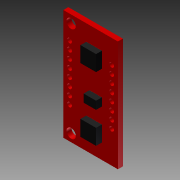
# Autodesk Inventor part: IMU
Saved by Autodesk Inventor 2012 (Build 160160000, 160)
## iProperties
Created: 2012-03-02
Part Number: IMU
Material: Default
Document SubType Name: Modeling
Designer: Lauszus
Density: 1 g/cm^3
Author: Lauszus
Autodesk Inventor part; units mm, degrees
ref_plane "YZ Plane" through (0, 0, 0) normal (1, 0, 0) x (0, 1, 0)
ref_plane "XZ Plane" through (0, 0, 0) normal (0, 1, 0) x (-1, 0, 0)
ref_plane "XY Plane" through (0, 0, 0) normal (0, 0, 1) x (1, 0, 0)
sketch "Sketch1" plane through (0, 0, 0) normal (0, 0, 1) x (1, 0, 0)
  line L0 (35.093, -7.2202) -> (-19.907, -7.2202)
  line L1 (-19.907, -7.2202) -> (-19.907, 74.7798)
  line L2 (-19.907, 74.7798) -> (35.093, 74.7798)
  line L3 (35.093, 74.7798) -> (35.093, -7.2202)
  line L4 (-1.6316, 73.7798) -> (15.8684, 73.7798)
  line L5 (15.8684, 73.7798) -> (15.8684, 38.2798)
  line L6 (15.8684, 38.2798) -> (-1.6316, 38.2798)
  line L7 (-1.6316, 38.2798) -> (-1.6316, 73.7798)
  circle A0 centre (7.5885, 28.2798) radius 5.75
  line L8 (12.233, 6.0025) -> (3.233, 6.0025)
  line L9 (3.233, 6.0025) -> (3.233, -3.9975)
  line L10 (3.233, -3.9975) -> (12.233, -3.9975)
  line L11 (12.233, -3.9975) -> (12.233, 6.0025)
  circle A1 centre (7.5885, 28.2798) radius 1.25
  line L12 (3.233, 6.0025) -> (-2.767, 6.0025)
  line L13 (-2.767, 6.0025) -> (-2.767, -3.9975)
  line L14 (-2.767, -3.9975) -> (3.233, -3.9975)
  line L15 (3.233, -3.9975) -> (3.233, 6.0025)
  line L16 (12.233, 5.3167) -> (16.7288, 5.3167)
  line L17 (16.7288, 5.3167) -> (16.7288, 2.7767)
  line L18 (16.7288, 2.7767) -> (12.233, 2.7767)
  line L19 (12.233, 2.7767) -> (12.233, 5.3167)
  line L20 (12.233, -1.5375) -> (12.233, 1.0025)
  line L21 (12.233, -3.4895) -> (12.233, -0.9495)
  line L22 (12.233, 2.2687) -> (16.7288, 2.2687)
  line L23 (16.7288, 2.2687) -> (16.7288, -0.2713)
  line L24 (16.7288, -0.2713) -> (12.233, -0.2713)
  line L25 (12.233, -0.2713) -> (12.233, 2.2687)
  line L26 (12.233, -0.7793) -> (16.7288, -0.7793)
  line L27 (16.7288, -0.7793) -> (16.7288, -3.3193)
  line L28 (16.7288, -3.3193) -> (12.233, -3.3193)
  line L29 (12.233, -3.3193) -> (12.233, -0.7793)
  circle A2 centre (0.233, 0.9987) radius 1.5
  circle A3 centre (0.3684, 66.2798) radius 0.75
  circle A4 centre (0.3684, 63.7398) radius 0.75
  circle A5 centre (0.3684, 61.1998) radius 0.75
  circle A6 centre (0.3684, 58.6598) radius 0.75
  circle A7 centre (0.3684, 56.1198) radius 0.75
  circle A8 centre (0.3684, 53.5798) radius 0.75
  circle A9 centre (0.3684, 51.0398) radius 0.75
  circle A10 centre (0.3684, 48.4998) radius 0.75
  circle A11 centre (13.8684, 63.7398) radius 0.75
  circle A12 centre (13.8684, 58.6598) radius 0.75
  circle A13 centre (13.8684, 56.1198) radius 0.75
  circle A14 centre (13.8684, 53.5798) radius 0.75
  circle A15 centre (13.8684, 48.4998) radius 0.75
  circle A16 centre (13.8684, 66.2798) radius 0.75
  circle A17 centre (13.8684, 51.0398) radius 0.75
  circle A18 centre (13.8684, 61.1998) radius 0.75
  line L30 (-17.907, 69.7798) -> (-16.407, 69.7798)
  line L31 (-16.407, 69.7798) -> (-16.407, -2.2202)
  line L32 (-16.407, -2.2202) -> (-17.907, -2.2202)
  line L33 (-17.907, -2.2202) -> (-17.907, 69.7798)
  line L34 (-15.367, -2.2202) -> (-13.867, -2.2202)
  line L35 (-13.867, -2.2202) -> (-13.867, 69.7798)
  line L36 (-13.867, 69.7798) -> (-15.367, 69.7798)
  line L37 (-15.367, 69.7798) -> (-15.367, -2.2202)
  line L38 (31.593, 69.7798) -> (33.093, 69.7798)
  line L39 (33.093, 69.7798) -> (33.093, -2.2202)
  line L40 (33.093, -2.2202) -> (31.593, -2.2202)
  line L41 (31.593, -2.2202) -> (31.593, 69.7798)
  line L42 (30.553, -2.2202) -> (29.053, -2.2202)
  line L43 (29.053, -2.2202) -> (29.053, 69.7798)
  line L44 (29.053, 69.7798) -> (30.553, 69.7798)
  line L45 (30.553, 69.7798) -> (30.553, -2.2202)
  line L46 (5.8684, 68.7798) -> (10.8684, 68.7798)
  line L47 (10.8684, 68.7798) -> (10.8684, 63.7798)
  line L48 (10.8684, 63.7798) -> (5.8684, 63.7798)
  line L49 (5.8684, 63.7798) -> (5.8684, 68.7798)
  line L50 (6.8684, 55.8198) -> (10.8684, 55.8198)
  line L51 (10.8684, 55.8198) -> (10.8684, 53.2798)
  line L52 (10.8684, 53.2798) -> (6.8684, 53.2798)
  line L53 (6.8684, 53.2798) -> (6.8684, 55.8198)
  line L54 (5.8684, 48.2798) -> (10.8684, 48.2798)
  line L55 (10.8684, 48.2798) -> (10.8684, 43.2798)
  line L56 (10.8684, 43.2798) -> (5.8684, 43.2798)
  line L57 (5.8684, 43.2798) -> (5.8684, 48.2798)
  circle A19 centre (0.8684, 71.2798) radius 1.5
  circle A20 centre (0.8684, 40.7798) radius 1.5
  point P0 (0, 0)
  point P1 (0, 0)
  dimension "d0" = 82
  dimension "d1" = 55
  dimension "d2" = 17.5
  dimension "d3" = 35.5
  dimension "d4" = 11.5
  dimension "d5" = 2.5
  dimension "d6" = 1
  dimension "d7" = 10
  dimension "d8" = 27.4955
  dimension "d9" = 9
  dimension "d10" = 10
  dimension "d11" = 6
  dimension "d12" = 22.86
  dimension "d13" = 19.2246
  dimension "d14" = 2.54
  dimension "d15" = 0.6858
  dimension "d16" = 10
  dimension "d17" = 2.54
  dimension "d18" = 0.508
  dimension "d19" = 4.4958
  dimension "d20" = 4.4958
  dimension "d21" = 2.54
  dimension "d22" = 4.4958
  dimension "d23" = 0.508
  dimension "d24" = 3
  dimension "d25" = 1.5
  dimension "d26" = 7.5
  dimension "d27" = 2
  dimension "d28" = 1.5
  dimension "d29" = 1.5
  dimension "d30" = 1.5
  dimension "d31" = 1.5
  dimension "d32" = 1.5
  dimension "d33" = 1.5
  dimension "d34" = 1.5
  dimension "d35" = 2.54
  dimension "d36" = 2.54
  dimension "d37" = 2.54
  dimension "d38" = 2.54
  dimension "d39" = 2.54
  dimension "d40" = 2.54
  dimension "d41" = 2.54
  dimension "d42" = 1.5
  dimension "d43" = 1.5
  dimension "d44" = 1.5
  dimension "d45" = 1.5
  dimension "d46" = 1.5
  dimension "d47" = 1.5
  dimension "d48" = 1.5
  dimension "d49" = 1.5
  dimension "d50" = 2.54
  dimension "d51" = 2.54
  dimension "d52" = 2.54
  dimension "d53" = 2.54
  dimension "d54" = 2.54
  dimension "d55" = 2.54
  dimension "d56" = 2.54
  dimension "d57" = 2
  dimension "d58" = 7.5
  dimension "d59" = 2
  dimension "d60" = 2
  dimension "d61" = 2
  dimension "d62" = 2
  dimension "d63" = 2
  constraints: 116 end point, 28 parallel, 21 centre point, 14 horizontal, 14 perpendicular, 4 point on line, 1 coincident, 1 midpoint
  measures "d0" distance of L0.end L1.end
  measures "d1" distance of L1.end L2.end
  measures "d2" distance of L4.start L4.end
  measures "d3" distance of L4.end L5.end
  measures "d4" diameter of A0
  measures "d5" diameter of A1
  measures "d6" distance between parallel lines of L2 L4
  measures "d7" distance from line of A0.centre L6
  measures "d8" distance from line of L1 A0.centre
  measures "d9" distance between parallel lines of L9 L11
  measures "d10" distance of L10.end L8.start
  measures "d11" distance of L8.end L12.end
  measures "d12" distance between parallel lines of L3 L11
  measures "d13" distance between parallel lines of L3 L5
  measures "d14" distance of L16.end L17.end
  measures "d15" distance between parallel lines of L8 L16
  measures "d16" distance of L14.end L8.end
  measures "d17" distance of L22.end L23.end
  measures "d18" distance between parallel lines of L18 L22
  measures "d19" distance of L16.start L16.end
  measures "d20" distance of L22.start L22.end
  measures "d21" distance of L26.end L27.end
  measures "d22" distance of L26.start L26.end
  measures "d23" distance between parallel lines of L24 L26
  measures "d24" diameter of A2
  measures "d25" diameter of A3
  measures "d26" distance from line of L4 A3.centre
  measures "d27" distance from line of L7 A3.centre
  measures "d28" diameter of A4
  measures "d29" diameter of A5
  measures "d30" diameter of A6
  measures "d31" diameter of A7
  measures "d32" diameter of A8
  measures "d33" diameter of A9
  measures "d34" diameter of A10
  measures "d35" distance of A4.centre A3.centre
  measures "d36" distance between centres of A5 A4
  measures "d37" distance between centres of A6 A5
  measures "d38" distance of A7.centre A6.centre
  measures "d39" distance between centres of A8 A7
  measures "d40" distance between centres of A9 A8
  measures "d41" distance between centres of A10 A9
  measures "d42" diameter of A16
  measures "d43" diameter of A11
  measures "d44" diameter of A18
  measures "d45" diameter of A12
  measures "d46" diameter of A13
  measures "d47" diameter of A14
  measures "d48" diameter of A17
  measures "d49" diameter of A15
  measures "d50" distance of A11.centre A16.centre
  measures "d51" distance between centres of A18 A11
  measures "d52" distance between centres of A12 A18
  measures "d53" distance of A13.centre A12.centre
  measures "d54" distance between centres of A14 A13
  measures "d55" distance between centres of A17 A14
  measures "d56" distance between centres of A15 A17
  measures "d57" distance from line of L5 A16.centre
  measures "d58" distance from line of L4 A16.centre
  measures "d59" distance from line of L5 A11.centre
  measures "d60" distance from line of L5 A18.centre
  measures "d61" distance from line of L5 A12.centre
  measures "d62" distance from line of L5 A13.centre
  measures "d63" distance from line of L5 A14.centre
extrude "Extrusion1" add sketch "Sketch1" along normal blind 2 contours L46 L47 L48 L49 | L50 L51 L52 L53 | L54 L55 L56 L57
fillet "Fillet1" radius 0.127 12 edges at (8.3684, 68.7798, 0) (5.8684, 66.2798, 0) (8.3684, 63.7798, 0) (10.8684, 66.2798, 0) (6.8684, 54.5498, 0) (8.8684, 55.8198, 0) (10.8684, 54.5498, 0) (8.8684, 53.2798, 0) (8.3684, 48.2798, 0) (5.8684, 45.7798, 0) (8.3684, 43.2798, 0) (10.8684, 45.7798, 0)
extrude "Extrusion2" add sketch "Sketch1" against normal blind 1.6 contours L4 L5 L6 L7 | L46 L47 L48 L49 | L50 L51 L52 L53 | L54 L55 L56 L57
body "Solid1"
